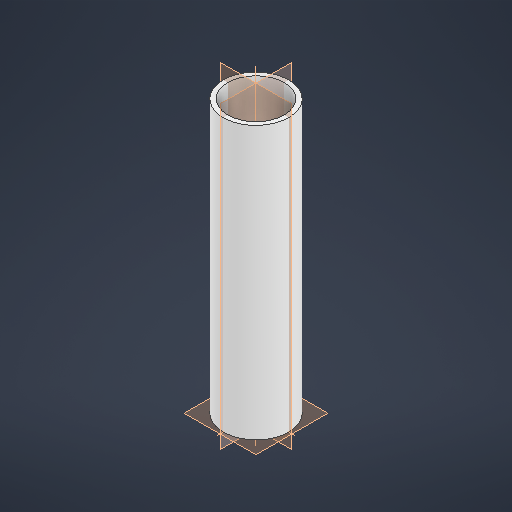
# Autodesk Inventor part: m12-rings
Saved by Autodesk Inventor 2026.1 (Build 301233020, 233B)
## iProperties
Created: 2025-03-19
Part Number: m12-rings
Material: PET Plastic
Document SubType Name: Modeling
Designer: yehorderehus
Density: 1.541 g/cm^3
Appearance: Smooth - White
Author: yehorderehus
Autodesk Inventor part; units mm, degrees
sketch "Sketch1" plane through (0, 0, 0) normal (0, 1, 0) x (-1, 0, 0)
  circle A0 centre (0, 0) radius 6.2
  circle A1 centre (0, 0) radius 7.2
  dimension "d0" = 12.4
  dimension "d1" = 1
  constraints: 2 centre point, 2 coincident
  measures "d0" diameter of A0
  measures "d1" radial gap between concentric circles of A0 A1
extrude "Extrusion1" add sketch "Sketch1" along normal blind 60
body "Solid1"
